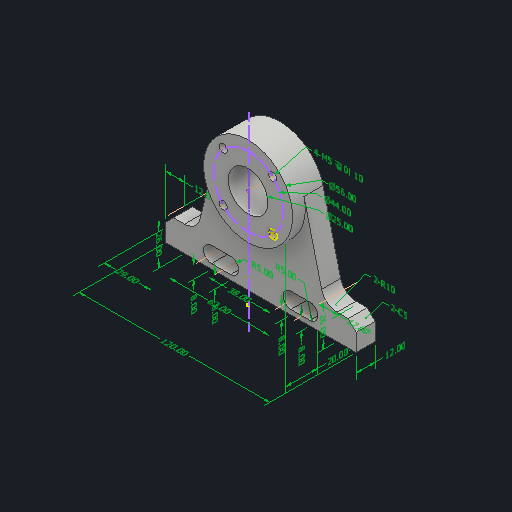
# Autodesk Inventor part: 아이들러 풀리 브라켓
Saved by Autodesk Inventor 2027.1 (Build 311270010, 270A)
## iProperties
Created: 2026-08-22
Part Number: 아이들러 풀리 브라켓
Material: 일반
Document SubType Name: Modeling
Designer: 202502
Density: 1 g/cm^3
Appearance: 기본값
Author: 202502
Autodesk Inventor part; units mm, degrees
ref_plane "YZ Plane" through (0, 0, 0) normal (1, 0, 0) x (0, 1, 0)
ref_plane "XZ Plane" through (0, 0, 0) normal (0, 1, 0) x (-1, 0, 0)
ref_plane "XY Plane" through (0, 0, 0) normal (0, 0, 1) x (1, 0, 0)
sketch "스케치1" plane through (0, 0, 0) normal (0, 0, 1) x (1, 0, 0)
  line L0 (-60, 0) -> (60, 0)
  line L1 (60, 0) -> (60, 62)
  line L2 (-60, 62) -> (-60, 0)
  line L3 (0, 0) -> (0, 151.2751)
  arc A0 (-31, 13) -> (-31, 3) centre (-31, 8) ccw
  arc A1 (-19, 3) -> (-19, 13) centre (-19, 8) ccw
  line L4 (-31, 13) -> (-19, 13)
  line L5 (-31, 3) -> (-19, 3)
  arc A2 (31, 3) -> (31, 13) centre (31, 8) ccw
  arc A3 (19, 13) -> (19, 3) centre (19, 8) ccw
  line L6 (31, 13) -> (19, 13)
  line L7 (31, 3) -> (19, 3)
  arc A4 (28, 62) -> (-28, 62) centre (0, 62) ccw
  line L8 (60, 62) -> (28, 62)
  line L9 (-28, 62) -> (-60, 62)
  dimension "d0" = 120
  dimension "d1" = 62
  dimension "d2" = 29
  dimension "d3" = 10
  dimension "d5" = 10
  dimension "d6" = 12
  dimension "d7" = 56
  dimension "d8" = 8
  constraints: 20 end point, 10 point on circle, 6 symmetric about line, 5 centre point, 4 parallel, 1 horizontal, 1 midpoint, 1 perpendicular, 1 point on line, 1 tangent, 1 vertical, 3 other
  measures "d0" distance of L1.end L2.start
  measures "d1" distance of L0.end L1.end
  measures "d2" distance from line of L2 A0.centre
  measures "d3" diameter of A0
  measures "d5" diameter of A1
  measures "d6" distance of A0.centre A1.centre
  measures "d7" diameter of A4
  measures "d8" distance from line of L0 A0.centre
extrude "돌출1" add sketch "스케치1" along normal blind 12
sketch "스케치2" plane through (0, 0, 12) normal (0, 0, 1) x (1, 0, 0)
  circle A0 centre (0, 62) radius 28
  arc A1 (28, 62) -> (-28, 62) centre (0, 62) ccw projected
  point P0 (0, 0)
  dimension "d11" = 56
  constraints: 1 centre point, 1 concentric
  measures "d11" diameter of A0
extrude "돌출2" add sketch "스케치2" along normal blind 8
sketch "스케치3" plane through (0, 0, 12) normal (0, 0, 1) x (1, 0, 0)
  arc A0 (-48, 16) -> (-48, 36) centre (-48, 26) ccw
  line L0 (-48, 16) -> (-80.7935, 16)
  line L1 (-80.7935, 16) -> (-80.7935, 63.6006)
  line L2 (-80.7935, 63.6006) -> (-48, 63.6006)
  line L3 (-48, 63.6006) -> (-48, 36)
  line L4 (-60, 0) -> (60, 0) projected
  line L5 (-60, 62) -> (-60, 0) projected
  point P0 (0, 0)
  dimension "d14" = 20
  dimension "d15" = 16
  dimension "d16" = 12
  constraints: 8 end point, 2 parallel, 2 point on circle, 1 centre point, 1 horizontal, 1 perpendicular, 1 tangent
  measures "d14" diameter of A0
  measures "d15" distance between parallel lines of L4 L0
  measures "d16" distance from line of L5 A0.centre
extrude "돌출3" cut sketch "스케치3" against normal blind 20
mirror "미러1" about plane through (0, 0, 0) normal (1, 0, 0) of "돌출3"
chamfer "모따기1" distance 5 angle 45 2 edges at (-60, 16, 6) (60, 16, 6)
sketch "스케치4" plane through (0, 0, 12) normal (0, 0, 1) x (1, 0, 0)
  line L0 (-38.2901, 23.609) -> (-27.1878, 68.6949)
  circle A0 centre (0, 62) radius 28 projected
  arc A1 (-48, 16) -> (-48, 36) centre (-48, 26) ccw projected
  line L1 (0, 0) -> (0, 106.1688)
  line L2 (27.1878, 68.6949) -> (38.2901, 23.609)
  arc A2 (48, 36) -> (48, 16) centre (48, 26) ccw projected
  line L3 (-48, 16) -> (-74.8883, 57.476)
  line L4 (-74.8883, 57.476) -> (-15.255, 104.9361)
  line L5 (-15.255, 104.9361) -> (38.38, 97.6952)
  line L6 (38.38, 97.6952) -> (82.1306, 43.6078)
  line L7 (82.1306, 43.6078) -> (48, 16)
  constraints: 16 end point, 4 point on circle, 4 tangent, 1 perpendicular, 1 vertical
extrude "돌출4" cut sketch "스케치4" against normal blind 20 contours A1 L3 L4 L5 L1 A0 L0 | L1 L5 L6 L7 A2 L2 A0
sketch "스케치5" plane through (0, 0, 12) normal (0, 0, 1) x (1, 0, 0)
  line L0 (-38.2901, 23.609) -> (-28.8364, 62) projected
  line L1 (28.8364, 62) -> (28, 62) projected
  line L2 (28.8364, 62) -> (27.1878, 68.6949)
  line L3 (-27.1878, 68.6949) -> (-28.8364, 62)
  circle A0 centre (0, 62) radius 28 projected
  line L4 (-28.8364, 62) -> (-28, 62)
  line L5 (28, 62) -> (28.8364, 62)
  point P0 (0, 0)
  constraints: 8 end point, 4 point on circle, 2 horizontal, 2 tangent
extrude "돌출5" add sketch "스케치5" against normal blind 12 contours L1 A0 L2 | L4 L3 A0
sketch "스케치6" plane through (0, 62, 20) normal (0, 0, 1) x (1, 0, 0)
  circle A0 centre (0, 0) radius 12.5
  circle A1 centre (0, 0) radius 22
  circle A2 centre (15.5563, 15.5563) radius 2.5
  line L0 (-28.2851, -28.2851) -> (32.9008, 32.9008)
  line L1 (-49.5291, 0) -> (47.7327, 0)
  circle A3 centre (0, 0) radius 28 projected
  circle A4 centre (-15.5563, 15.5563) radius 2.5
  circle A5 centre (-15.5563, -15.5563) radius 2.5
  circle A6 centre (15.5563, -15.5563) radius 2.5
  point P0 (0, -62)
  dimension "d29" = 44
  dimension "d26" = 45
  dimension "d27" = 5
  dimension "d28" = 25
  dimension "d32" = 360
  constraints: 5 centre point, 4 end point, 3 point on line, 1 coincident, 1 concentric, 1 horizontal, 12 other
  measures "d26" angle of L0 L1
  measures "d27" diameter of A2
  measures "d28" diameter of A0
extrude "돌출6" cut sketch "스케치6" against normal blind 20 contours L1 L0 A0 | A0 L0 L1 | L0 L1 A0 | A0 L1 L0
extrude "돌출7" cut sketch "스케치6" against normal blind 10 contours L0 A1 A2 | A2 A1 L0 | A5 A1 L0 | L0 A1 A5 | A1 L0 A2 | A6 A1 | A1 A6 | A2 L0 A1 | L0 A5 A1 | A1 A5 L0 | A4 A1 | A1 A4
sketch "스케치7" plane through (0, 62, 20) normal (0, 0, 1) x (1, 0, 0)
  circle A0 centre (15.5563, -15.5563) radius 2.5 projected
  circle A1 centre (0, 0) radius 22
  line L0 (0, -76.267) -> (0, 43.2176)
  point P0 (0, -62)
  constraints: 2 end point, 1 vertical, 3 other
